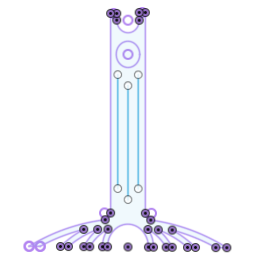
EAS Stand Sides (Autodesk Fusion 360 design; units mm, degrees)
Autodesk Fusion 360 part; units mm, degrees
note: some values were not read from the file. Set by a fixed rule: which sketch regions a step uses.
sketch "Main Body" plane through (0, 0, 0) normal (0, 0, 1) x (1, 0, 0)
  circle A0 centre (0, 0) radius 100
  circle A1 centre (0, 0) radius 95
  circle A2 centre (0, 25) radius 75
  circle A3 centre (0, 25) radius 70
  circle A4 centre (0, 50) radius 50
  circle A5 centre (0, 50) radius 45
  circle A6 centre (0, 75) radius 25
  circle A7 centre (0, 75) radius 20
  line L0 (-100, 75) -> (100, 75)
  circle A8 centre (0, 244.05) radius 7.5
  circle A9 centre (0, 244.05) radius 11.5
  line L1 (17, 96.1763) -> (-17, 96.1763)
  line L2 (-17, 96.1763) -> (-17, 200)
  line L3 (17, 200) -> (17, 96.1763)
  line L4 (17, 96.1763) -> (-17, 244.8247) construction
  line L5 (-17, 96.1763) -> (17, 244.8247) construction
  circle A10 centre (-23, 104.712) radius 6
  circle A11 centre (0, 274.05) radius 11
  line L6 (-17, 244.8247) -> (-11.4739, 244.8247)
  line L7 (-11, 247.4041) -> (-11, 279.8747)
  line L8 (-14, 282.8747) -> (-14, 282.8747)
  line L9 (-17, 279.8747) -> (-17, 244.8247)
  line L10 (17, 244.8247) -> (11.4739, 244.8247)
  line L11 (11, 247.4041) -> (11, 280.8747)
  line L12 (14, 283.8747) -> (14, 283.8747)
  line L13 (17, 280.8747) -> (17, 244.8247)
  circle A12 centre (0, -100) radius 200
  circle A13 centre (0, -100) radius 195
  circle A14 centre (23, 104.712) radius 6
  arc A15 (-14, 282.8747) -> (-17, 279.8747) centre (-14, 279.8747) ccw
  arc A16 (-11, 279.8747) -> (-14, 282.8747) centre (-14, 279.8747) ccw
  arc A17 (14, 283.8747) -> (11, 280.8747) centre (14, 280.8747) ccw
  arc A18 (17, 280.8747) -> (14, 283.8747) centre (14, 280.8747) ccw
  line L14 (-17, 200) -> (-17, 244.8247)
  line L15 (17, 244.8247) -> (17, 200)
  line L16 (-17, 244.8247) -> (-11.4739, 244.8247)
  line L17 (11.4739, 244.8247) -> (17, 244.8247)
  point P0 (0, 170.5005)
  point P1 (-17, 264.8247)
  point P2 (17, 264.8247)
  dimension "d1" = 200
  dimension "d2" = 190
  dimension "d3" = 150
  dimension "d4" = 140
  dimension "d5" = 100
  dimension "d6" = 90
  dimension "d7" = 50
  dimension "d8" = 40
  dimension "d11" = 15
  dimension "d12" = 23
  dimension "d13" = 34
  dimension "d15" = 12
  dimension "d16" = 22
  dimension "d17" = 20
  dimension "d19" = 20
  dimension "d23" = 400
  dimension "d24" = 390
  dimension "d25" = 12
  dimension "d26" = 3
  dimension "d27" = 3
  dimension "d28" = 3
  dimension "d29" = 3
  constraint coincident A0.centre A1.centre
  constraint horizontal L0
  constraint concentric A8 A9
  constraint perpendicular L1 L2
  constraint parallel L1 L16
  constraint parallel L2 L3
  constraint horizontal L1
  constraint coincident L4 P0
  constraint coincident L5 P0
  constraint tangent L2 A10
  constraint horizontal L6
  constraint vertical L7
  constraint vertical L9
  constraint horizontal L10
  constraint vertical L11
  constraint vertical L13
  constraint tangent L3 A14
  constraint tangent A12 A14
  constraint tangent A10 A12
  constraint coincident P1 L9
  constraint tangent L9 A15
  constraint tangent L7 A16
  constraint tangent L11 A17
  constraint coincident P2 L12
  constraint coincident P2 L13
  constraint tangent L13 A18
  constraint perpendicular L1 L14
  constraint parallel L2 L15
  constraint coincident A9 L7.start
  constraint coincident A9 L11.start
  constraint coincident A9 L10.end
  constraint collinear L16 L17
  constraint coincident A9 L6.end
  measures "d1" diameter of A0
  measures "d2" diameter of A1
  measures "d3" diameter of A2
  measures "d4" diameter of A3
  measures "d5" diameter of A4
  measures "d6" diameter of A5
  measures "d7" diameter of A6
  measures "d8" diameter of A7
  measures "d11" diameter of A8
  measures "d12" diameter of A9
  measures "d13" distance of L4.end L5.end
  measures "d15" diameter of A10
  measures "d16" diameter of A11
  measures "d17" distance of L4.end P1
  measures "d19" distance of L5.end P2
  measures "d23" diameter of A12
  measures "d24" diameter of A13
  measures "d25" diameter of A14
  measures "d26" radius of A15
  measures "d27" radius of A16
  measures "d28" radius of A17
  measures "d29" radius of A18
extrude "Extrude1" add sketch "Main Body" along normal blind 16 contours A0 A1 A2 L0 A13 | A0 A1 A2 L0 A13 | A0 A2 L3 A13 | A0 L0 L3 A12 A13 | A0 L0 L2 A12 A13 | A0 A2 L2 A13 | A0 A2 L3 | A0 L3 A12 | A2 A4 L3 A13 | A1 A2 A4 A13 | A0 L2 A12 | A0 A2 L2 | A1 A2 A4 A13 | A2 A4 L2 A13 | A2 A4 L2 | A2 A4 L3 | A4 A6 L1 L2 | A4 A6 L1 L3 | A6 L1 | A9 L2 L3 L6 L10 A12 L14 L15 L16 L17 | L3 A12 A14 | A4 A6 L1 L3 A13 | A1 A4 A6 A13 | A1 A3 A4 A6 | L2 A10 A12 | A1 A4 A6 A13 | A4 A6 L1 L2 A13 | A1 A3 A4 A6 | A6 L1 A13 | A1 A6 A13 | A1 A3 A6 | A3 A4 A5 A6 L0 | A1 A6 A13 | A1 A3 A6 | A3 A4 A5 A6 L0 | A3 A5 A6 | A3 A5 A6 | A5 A6 A7 L0 | A5 A6 A7 L0 | A9 L10 L11 L13 A17 A18 L17 | A9 L6 L7 L9 A15 A16 L16 | A9 A11 L7 L11
extrude "Extrude3" add sketch "Main Body" along normal blind 8 contours A9
sketch "Design Lines" plane through (0, 0, 16) normal (0, 0, 1) x (1, 0, 0)
  line L0 (0, 216.55) -> (0, 116.55)
  line L1 (-10, 126.15) -> (-10, 226.15)
  line L2 (10, 126.15) -> (10, 226.15)
  arc A0 (86.0233, 75) -> (43.3299, 90.125) centre (0, -100) ccw
  line L3 (-96.8246, 75) -> (-86.0233, 75)
  arc A1 (-22.3301, 98.7495) -> (-96.8246, 75) centre (0, -100) ccw
  arc A2 (-43.3299, 90.125) -> (-86.0233, 75) centre (0, -100) ccw
  arc A3 (-43.3299, 90.125) -> (-66.1438, 75) centre (0, 0) ccw
  line L4 (-66.1438, 75) -> (-58.3095, 75)
  arc A4 (-29.6637, 90.25) -> (-58.3095, 75) centre (0, 0) ccw
  arc A5 (-29.6637, 90.25) -> (-43.3013, 75) centre (0, 50) ccw
  line L5 (-43.3013, 75) -> (-37.4166, 75)
  arc A6 (-19.615, 90.5) -> (-37.4166, 75) centre (0, 50) ccw
  arc A7 (-19.615, 90.5) -> (-25, 75) centre (0, 75) ccw
  line L6 (-25, 75) -> (-20, 75)
  arc A8 (20, 75) -> (-20, 75) centre (0, 75) ccw
  arc A9 (25, 75) -> (19.615, 90.5) centre (0, 75) ccw
  arc A10 (37.4166, 75) -> (19.615, 90.5) centre (0, 50) ccw
  line L7 (37.4166, 75) -> (43.3013, 75)
  circle A11 centre (0, 244.05) radius 11.5
  arc A12 (17, 280.8747) -> (11, 280.8747) centre (14, 280.8747) ccw
  line L8 (11, 280.8747) -> (11, 274.05)
  arc A13 (-11, 274.05) -> (11, 274.05) centre (0, 274.05) ccw
  line L9 (-11, 274.05) -> (-11, 279.8747)
  arc A14 (-11, 279.8747) -> (-17, 279.8747) centre (-14, 279.8747) ccw
  line L10 (-17, 279.8747) -> (-17, 104.712)
  arc A15 (-22.3301, 98.7495) -> (-17, 104.712) centre (-23, 104.712) ccw
  line L11 (20, 75) -> (25, 75)
  arc A16 (43.3013, 75) -> (29.6637, 90.25) centre (0, 50) ccw
  arc A17 (58.3095, 75) -> (29.6637, 90.25) centre (0, 0) ccw
  line L12 (58.3095, 75) -> (66.1438, 75)
  arc A18 (66.1438, 75) -> (43.3299, 90.125) centre (0, 0) ccw
  line L13 (86.0233, 75) -> (96.8246, 75)
  arc A19 (96.8246, 75) -> (22.3301, 98.7495) centre (0, -100) ccw
  arc A20 (17, 104.712) -> (22.3301, 98.7495) centre (23, 104.712) ccw
  line L14 (17, 104.712) -> (17, 280.8747)
  constraint parallel L0 L1
